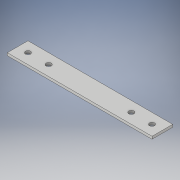
# Autodesk Inventor part: plate 1
Saved by Autodesk Inventor 2017 (Build 210142000, 142)
## iProperties
Created: 2018-07-12
Part Number: plate 1
Material: Generic
Document SubType Name: Modeling
Designer: sinner
Density: 1 g/cm^3
Appearance: Default
Author: sinner
Autodesk Inventor part; units mm, degrees
ref_plane "YZ Plane" through (0, 0, 0) normal (1, 0, 0) x (0, 1, 0)
ref_plane "XZ Plane" through (0, 0, 0) normal (0, 1, 0) x (-1, 0, 0)
ref_plane "XY Plane" through (0, 0, 0) normal (0, 0, 1) x (1, 0, 0)
sketch "Sketch1" plane through (0, 0, 0) normal (1, 0, 0) x (0, 1, 0)
  line L0 (0, 0) -> (3.175, 0)
  line L1 (3.175, 0) -> (3.175, -25.4)
  line L2 (3.175, -25.4) -> (0, -25.4)
  line L3 (0, -25.4) -> (0, 0)
  dimension "d0" = 3.175
  dimension "d1" = 25.4
  constraints: 8 end point, 2 parallel, 1 horizontal, 1 perpendicular
  measures "d0" distance of L1.end L2.end
  measures "d1" distance of L0.end L1.end
extrude "Extrusion1" add sketch "Sketch1" along normal blind 177.8
sketch "Sketch2" plane through (0, 3.175, 0) normal (0, 1, 0) x (1, 0, 0)
  line L0 (0, 25.4) -> (0, 0) projected
  line L1 (0, 12.7) -> (106.9215, 12.7) construction
  circle A0 centre (12.7, 12.7) radius 3.175
  line L2 (0, 25.4) -> (177.8, 25.4) projected
  line L3 (88.9, 25.4) -> (88.9, 2.1168) construction
  circle A1 centre (38.1, 12.7) radius 3.175
  circle A2 centre (165.1, 12.7) radius 3.175
  circle A3 centre (139.7, 12.7) radius 3.175
  dimension "d4" = 6.35
  dimension "d5" = 50.8
  dimension "d6" = 76.2
  constraints: 4 centre point, 4 end point, 2 midpoint, 2 point on line, 2 symmetric about line, 1 equal radius, 1 horizontal, 1 vertical, 2 other
  measures "d4" diameter of A0
  measures "d5" distance from line of L3 A1.centre
  measures "d6" distance from line of L3 A0.centre
extrude "Extrusion2" cut sketch "Sketch2" against normal blind 3.175
body "Solid1"
